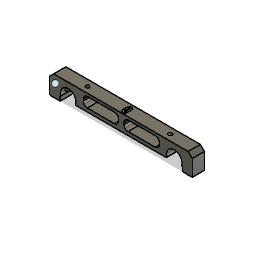
ERCF Reprack Mount (Autodesk Fusion 360 design; units mm, degrees)
Autodesk Fusion 360 part; units mm, degrees
sketch "Sketch1" plane through (0, -7, 0) normal (0, -1, 0) x (1, 0, 0)
  line L0 (51.9203, 0.4) -> (56.186, 4.6657)
  line L1 (56.186, 4.6657) -> (56.186, 10.3343)
  line L2 (56.186, 10.3343) -> (51.9203, 14.6)
  line L3 (51.9203, 14.6) -> (7, 14.6)
  line L4 (7, 14.6) -> (7, 0.4)
  line L5 (7, 0.4) -> (51.9203, 0.4)
  circle A0 centre (50.586, 7.5) radius 2.1
  line L6 (-95, 25, 0.3) -> (120, 25, 0.3)
  line L7 (120, 25, 0.3) -> (120, -10, 0.3)
  line L8 (120, -10, 0.3) -> (-95, -10, 0.3)
  line L9 (-95, -10, 0.3) -> (-95, 25, 0.3)
extrude "Extrude1" add sketch "Sketch1" along normal blind 20 contours L6 L7 L8 L9 in plane through (0, -7.3, 0) normal (0, -1, 0)
hole "Hole1" at (-67.2267, -23.4953, 25) direction (0, 0, -1) diameter 19 depth 40 tip angle 118
hole "Hole2" at (63.0011, -23.5949, 25) direction (0, 0, -1) diameter 19 depth 40 tip angle 118
fillet "Fillet1" radius 0.75 4 edges at (54.2534, -27.3, 7.5) (-75.9315, -27.3, 7.5) (71.7488, -27.3, 7.5) (-58.5219, -27.3, 7.5)
extrude "Extrude2" cut 1 faces at (120, -20.6333, 13.3333) along direction (-1, 0, 0) blind 25
sketch "Sketch2" plane through (-95, 0, 0) normal (-1, 0, 0) x (0, 0, 1)
  line L0 (25, -7.3) -> (-10, -7.3)
  line L1 (-10, -7.3) -> (-10, -27.3)
  line L2 (-10, -27.3) -> (25, -27.3)
  line L3 (25, -27.3) -> (25, -7.3)
extrude "Extrude3" cut sketch "Sketch2" against normal blind 5
chamfer "Chamfer1" distance 5 angle 45 1 edges at (-90, -7.3, 7.5)
extrude "Extrude4" cut 1 faces at (95, -20.6333, 13.3333) along direction (-1, 0, 0) blind 10
chamfer "Chamfer2" distance 5 angle 45 1 edges at (85, -7.3, 7.5)
sketch "Sketch3" plane through (0, 0, -10) normal (0, 0, -1) x (-1, 0, 0)
  line L0 (-80, -7.3) -> (-85, -12.3)
  line L1 (-85, -12.3) -> (-85, -27.3)
  line L2 (-85, -27.3) -> (-72.8159, -27.3)
  arc A0 (-72.8159, -27.3) -> (-72.0977, -26.3338) centre (-72.8159, -26.55) ccw
  arc A1 (-53.9045, -26.3338) -> (-72.0977, -26.3338) centre (-63.0011, -23.5949) ccw
  arc A2 (-53.9045, -26.3338) -> (-53.1863, -27.3) centre (-53.1863, -26.55) ccw
  line L3 (-53.1863, -27.3) -> (57.4425, -27.3)
  arc A3 (57.4425, -27.3) -> (58.1584, -26.3265) centre (57.4425, -26.55) ccw
  arc A4 (76.295, -26.3265) -> (58.1584, -26.3265) centre (67.2267, -23.4953) ccw
  arc A5 (76.295, -26.3265) -> (77.0109, -27.3) centre (77.0109, -26.55) ccw
  line L4 (77.0109, -27.3) -> (90, -27.3)
  line L5 (90, -27.3) -> (90, -12.3)
  line L6 (90, -12.3) -> (85, -7.3)
  line L7 (85, -7.3) -> (-80, -7.3)
  line L8 (-44.6269, -10.674) -> (-1.3009, -10.674)
  line L9 (-1.3009, -10.674) -> (-1.3009, -22.9741)
  line L10 (-1.3009, -22.9741) -> (-44.6269, -22.9741)
  line L11 (-44.6269, -22.9741) -> (-44.6269, -10.674)
  line L12 (48.6991, -22.9741) -> (5.3731, -22.9741)
  line L13 (5.3731, -22.9741) -> (5.3731, -10.674)
  line L14 (5.3731, -10.674) -> (48.6991, -10.674)
  line L15 (48.6991, -10.674) -> (48.6991, -22.9741)
  constraint horizontal L8
  constraint vertical L9
  constraint horizontal L10
  constraint vertical L11
  constraint horizontal L14
  constraint vertical L15
  constraint horizontal L12
  constraint vertical L13
extrude "Extrude5" cut sketch "Sketch3" against normal blind 110 contours L8 L9 L10 L11 | L12 L13 L14 L15
fillet "Fillet2" radius 5 8 edges at (44.6269, -22.9741, 7.5) (-5.3731, -22.9741, 7.5) (-48.6991, -22.9741, 7.5) (1.3009, -22.9741, 7.5) (1.3009, -10.674, 7.5) (-48.6991, -10.674, 7.5) (-5.3731, -10.674, 7.5) (44.6269, -10.674, 7.5)
sketch "Sketch4" plane through (0, -7.3, 0) normal (0, 1, 0) x (-1, 0, 0)
  line L0 (-80, 25) -> (-80, -10)
  line L1 (-80, -10) -> (85, -10)
  line L2 (85, -10) -> (85, 25)
  line L3 (85, 25) -> (-80, 25)
  circle A0 centre (-50.6018, 7.4858) radius 2.35
  dimension "d28" = 4.7
  measures "d28" diameter of A0
extrude "Extrude6" cut sketch "Sketch4" against normal blind 5.1 contours A0
sketch "Sketch5" plane through (0, -7.3, 0) normal (0, 1, 0) x (-1, 0, 0)
  circle A0 centre (-50.6018, 7.4858) radius 2.35
  line L0 (-80, 25) -> (-80, -10)
  line L1 (-80, -10) -> (85, -10)
  line L2 (85, -10) -> (85, 25)
  line L3 (85, 25) -> (-80, 25)
  circle A1 centre (50.6, 7.5) radius 2.35
  dimension "d31" = 4.7
  measures "d31" diameter of A1
extrude "Extrude7" cut sketch "Sketch5" against normal blind 5.2 contours A1
extrude "Extrude8" cut 1 faces at (-85.5414, -20.5679, -10) along direction (0, 0, 1) blind 10
extrude "Extrude9" cut 1 faces at (-85.5414, -20.5679, 25) along direction (0, 0, -1) blind 10
sketch "Sketch6" plane through (0, -7.3, 0) normal (0, 1, 0) x (-1, 0, 0)
  circle A0 centre (-50.6018, 7.4858) radius 2.35
  circle A1 centre (50.6, 7.5) radius 2.35
  line L0 (85, 15) -> (-80, 15)
  line L1 (-80, 15) -> (-80, 0)
  line L2 (-80, 0) -> (85, 0)
  line L3 (85, 0) -> (85, 15)
  line L4 (44.0725, 12.4652) -> (-40.5738, 12.4652) construction
  line L5 (-40.5738, 12.4652) -> (-40.5738, 3.1889) construction
  line L6 (-40.5738, 3.1889) -> (44.0725, 3.1889) construction
  line L7 (44.0725, 3.1889) -> (44.0725, 12.4652) construction
  dimension "d38" = 10
  text T0 "Q" font "Impact" height 10 align centre middle in box 84.6463 x 9.2763 at (44.0725, 12.4652) x (-1, 0) y (0, -1) spacing 1 kerned
extrude "Extrude10" cut sketch "Sketch6" against normal blind 0.5 text T0
sketch "sketch 2281" plane through (-90, -64.5442, -0.0498) normal (-1, 0, 0) x (0, 0, 1)
  circle A0 centre (8, 41) radius 2.35
extrude "Extrude11" cut sketch "sketch 2281" against normal blind 5
sketch "sketch 2294" plane through (-90, -64.5442, -0.0498) normal (-1, 0, 0) x (0, 0, 1)
  circle A0 centre (8, 41) radius 1.6
extrude "Extrude12" cut sketch "sketch 2294" against normal blind 32
sketch "sketch 2306" plane through (-90.2961, -64.7714, -0.0538) normal (-1, 0, 0) x (0, 0, 1)
  circle A0 centre (8, 41) radius 1.6
  circle A1 centre (8, 41) radius 2.35
extrude "Extrude13" cut sketch "sketch 2306" against normal blind 5.2
extrude "Extrude14" add 2 faces at (-85.6703, -27.3, 5) (76.8772, -27.3, 10) along direction (0, -1, 0) blind 5
